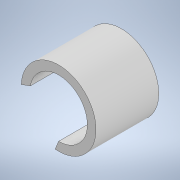
# Autodesk Inventor part: GuardTest
Saved by Autodesk Inventor 2020 (Build 240168000, 168)
## iProperties
Created: 2023-01-16
Part Number: GuardTest
Material: Generic
Document SubType Name: Modeling
Designer: agraa4529
Density: 1 g/cm^3
Appearance: Default
Author: agraa4529
Autodesk Inventor part; units mm, degrees
ref_plane "YZ Plane" through (0, 0, 0) normal (1, 0, 0) x (0, 1, 0)
ref_plane "XZ Plane" through (0, 0, 0) normal (0, 1, 0) x (-1, 0, 0)
ref_plane "XY Plane" through (0, 0, 0) normal (0, 0, 1) x (1, 0, 0)
sketch "Sketch1" plane through (0, 0, 0) normal (0, 0, 1) x (1, 0, 0)
  arc A0 (0, -4.125) -> (-4.0608, 0.7248) centre (0, 0) ccw
  line L0 (0, -4.125) -> (-4.0608, 0.7248)
  arc A1 (-0.4919, -5.3424) -> (-5.3588, 0.2578) centre (0, 0) ccw
  line L1 (0, -4.125) -> (-0.4919, -5.3424)
  line L2 (0, -4.125) -> (1.313, -4.125) construction
  line L3 (-4.0608, 0.7248) -> (-5.3588, 0.2578)
  dimension "d0" = 8.25
  dimension "d1" = 10.73
  dimension "d2" = 112
  constraints: 8 end point, 4 point on circle, 2 centre point, 2 coincident, 1 equal length, 1 horizontal
  measures "d0" diameter of A0
  measures "d1" diameter of A1
  measures "d2" angle of L1 L2
extrude "Extrusion1" add sketch "Sketch1" along normal blind 19 contours A0 L3 A1 L1
sketch "Sketch2" plane through (0, 0, 19) normal (0, 0, 1) x (1, 0, 0)
  arc A0 (-0.4919, -5.3424) -> (-5.3588, 0.2578) centre (0, 0) ccw projected
  line L0 (0, 5.365) -> (5.365, 0) construction
  line L1 (3.7936, 3.7936) -> (0, 5.365) construction
  line L2 (3.7936, 3.7936) -> (5.365, 0) construction
  line L3 (3.7936, 3.7936) -> (5.5269, 2.0604)
  line L4 (5.5269, 2.0604) -> (35.5269, 32.0604)
  line L5 (35.5269, 32.0604) -> (33.7936, 33.7936)
  line L6 (33.7936, 33.7936) -> (3.7936, 3.7936)
  line L7 (1.9965, 5.5907) -> (31.9965, 35.5907)
  line L8 (31.9965, 35.5907) -> (33.7936, 33.7936)
  line L9 (1.9965, 5.5907) -> (3.7936, 3.7936)
  line L10 (1.9965, 5.5907) -> (5.5269, 2.0604)
  line L11 (5.5269, 2.0604) -> (4.7391, 1.2726)
  line L12 (4.7391, 1.2726) -> (1.2088, 4.8029)
  line L13 (1.2088, 4.8029) -> (1.9965, 5.5907)
  line L14 (-3.7936, 3.7936) -> (-5.365, 0) construction
  line L15 (-3.7936, 3.7936) -> (-2.0604, 5.5269)
  line L16 (-2.0604, 5.5269) -> (-32.0604, 35.5269)
  line L17 (-32.0604, 35.5269) -> (-33.7936, 33.7936)
  line L18 (-33.7936, 33.7936) -> (-3.7936, 3.7936)
  line L19 (-5.5907, 1.9965) -> (-35.5907, 31.9965)
  line L20 (-35.5907, 31.9965) -> (-33.7936, 33.7936)
  line L21 (-5.5907, 1.9965) -> (-3.7936, 3.7936)
  line L22 (-5.5907, 1.9965) -> (-2.0604, 5.5269)
  line L23 (-2.0604, 5.5269) -> (-1.2726, 4.7391)
  line L24 (-1.2726, 4.7391) -> (-4.8029, 1.2088)
  line L25 (-4.8029, 1.2088) -> (-5.5907, 1.9965)
  line L26 (-3.7936, -3.7936) -> (0, -5.365) construction
  line L27 (-3.7936, -3.7936) -> (-5.5269, -2.0604)
  line L28 (-5.5269, -2.0604) -> (-35.5269, -32.0604)
  line L29 (-35.5269, -32.0604) -> (-33.7936, -33.7936)
  line L30 (-33.7936, -33.7936) -> (-3.7936, -3.7936)
  line L31 (-1.9965, -5.5907) -> (-31.9965, -35.5907)
  line L32 (-31.9965, -35.5907) -> (-33.7936, -33.7936)
  line L33 (-1.9965, -5.5907) -> (-3.7936, -3.7936)
  line L34 (-1.9965, -5.5907) -> (-5.5269, -2.0604)
  line L35 (-5.5269, -2.0604) -> (-4.7391, -1.2726)
  line L36 (-4.7391, -1.2726) -> (-1.2088, -4.8029)
  line L37 (-1.2088, -4.8029) -> (-1.9965, -5.5907)
  line L38 (3.7936, -3.7936) -> (5.365, 0) construction
  line L39 (3.7936, -3.7936) -> (2.0604, -5.5269)
  line L40 (2.0604, -5.5269) -> (32.0604, -35.5269)
  line L41 (32.0604, -35.5269) -> (33.7936, -33.7936)
  line L42 (33.7936, -33.7936) -> (3.7936, -3.7936)
  line L43 (5.5907, -1.9965) -> (35.5907, -31.9965)
  line L44 (35.5907, -31.9965) -> (33.7936, -33.7936)
  line L45 (5.5907, -1.9965) -> (3.7936, -3.7936)
  line L46 (5.5907, -1.9965) -> (2.0604, -5.5269)
  line L47 (2.0604, -5.5269) -> (1.2726, -4.7391)
  line L48 (1.2726, -4.7391) -> (4.8029, -1.2088)
  line L49 (4.8029, -1.2088) -> (5.5907, -1.9965)
  dimension "d5" = 30
  dimension "d6" = 30
  dimension "d11" = 360
  constraints: 100 end point, 4 parallel, 3 point on circle, 2 coincident, 2 collinear, 2 perpendicular, 2 tangent, 91 other
  measures "d5" horizontal distance of L5.end L1.start
  measures "d6" horizontal distance of L5.end L1.start
extrude "Extrusion2" add sketch "Sketch2" against normal blind 2 contours L47 L48 L49 A0 | A0 L39 L47 | L23 L24 L25 A0 | A0 L15 L23 | L11 L12 L13 A0 | A0 L3 L11 | L42 L41 L40 L39 | L45 L43 L44 L42 | A0 L49 L45 | L6 L5 L4 L3 | L9 L7 L8 L6 | A0 L13 L9 | L18 L17 L16 L15 | L21 L19 L20 L18 | A0 L25 L21
sketch "Sketch3" plane through (0, 0, 19) normal (0, 0, 1) x (1, 0, 0)
  circle A0 centre (0, 0) radius 47.75
  circle A1 centre (0, 0) radius 49.75
  dimension "d13" = 95.5
  dimension "d14" = 99.5
  constraints: 2 centre point, 2 coincident
  measures "d13" diameter of A0
  measures "d14" diameter of A1
extrude "Extrusion3" add sketch "Sketch3" against normal blind 2
sketch "Sketch4" plane through (0, 0, 19) normal (0, 0, 1) x (1, 0, 0)
  line L0 (-57.3156, 53.7161) -> (57.3156, 53.7161)
  line L1 (57.3156, 53.7161) -> (57.3156, -53.7161)
  line L2 (57.3156, -53.7161) -> (-57.3156, -53.7161)
  line L3 (-57.3156, -53.7161) -> (-57.3156, 53.7161)
  line L4 (-57.3156, 53.7161) -> (57.3156, -53.7161) construction
  line L5 (57.3156, 53.7161) -> (-57.3156, -53.7161) construction
  point P0 (0, 0)
  constraints: 12 end point, 2 midpoint, 2 parallel, 1 horizontal, 1 perpendicular
extrude "Extrusion4" cut sketch "Sketch4" against normal blind 10
body "Solid1"
